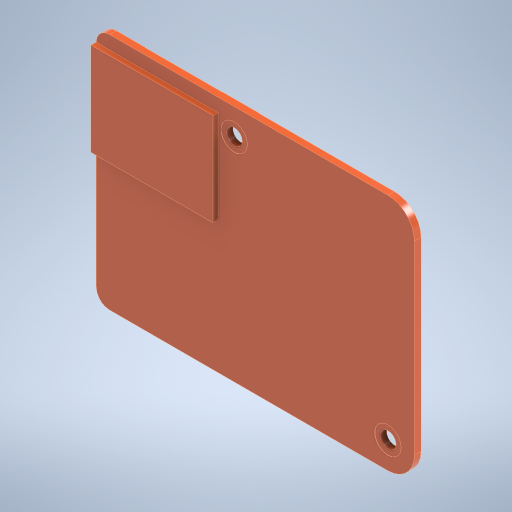
# Autodesk Inventor part: Part1
Saved by Autodesk Inventor 2023 (Build 270158000, 158)
## iProperties
Created: 2024-10-12
Part Number: Part1
Material: Phenolic Resin
Document SubType Name: Modeling
Designer: noname
Density: 1.38 g/cm^3
Appearance: Smooth - Light Orange
Mass: 5.00354 g
Surface Area: 57.0326 cm^2
Volume: 3.62576 cm^3
Author: noname
Autodesk Inventor part; units mm, degrees
ref_plane "YZ Plane" through (0, 0, 0) normal (1, 0, 0) x (0, 1, 0)
ref_plane "XZ Plane" through (0, 0, 0) normal (0, 1, 0) x (-1, 0, 0)
ref_plane "XY Plane" through (0, 0, 0) normal (0, 0, 1) x (1, 0, 0)
sketch "Sketch1" plane through (0, 0, 0) normal (0, 0, 1) x (1, 0, 0)
  line L0 (10.25, 20.1716) -> (10.25, 23.6716) projected
  line L1 (-1.25, 23.6716) -> (10.25, 23.6716) projected
  arc A0 (0.75, 23.3284) -> (-1.25, 23.6716) centre (-1.25, 17.6716) ccw projected
  line L2 (0.75, 23.3284) -> (0.75, -11.8284) projected
  arc A1 (-1.25, -13.8284) -> (0.75, -11.8284) centre (-1.25, -11.8284) ccw projected
  arc A2 (-1.25, -13.8284) -> (-4.75, -17.3284) centre (-1.25, -17.3284) ccw projected
  line L3 (-4.75, -17.3284) -> (-4.75, -23.3284) projected
  line L4 (10.25, -23.3284) -> (-4.75, -23.3284) projected
  line L5 (10.25, -23.3284) -> (10.25, -19.8284) projected
  line L6 (10.25, -19.8284) -> (6.75, -19.8284) projected
  line L7 (6.75, -19.8284) -> (6.75, 8.1716) projected
  line L8 (6.75, 8.1716) -> (16.75, 8.1716) projected
  line L9 (16.75, 17.1716) -> (16.75, 8.1716) projected
  line L10 (16.75, 17.1716) -> (13.25, 17.1716) projected
  arc A3 (10.25, 20.1716) -> (13.25, 17.1716) centre (13.25, 20.1716) ccw projected
  circle A4 centre (-1.25, -17.3284) radius 1.5 projected
  line L11 (-57.25, 4.6716) -> (-57.25, 20.1716) projected
  line L12 (-57.25, 4.6716) -> (-50.25, 4.6716) projected
  arc A5 (-50.25, 4.6716) -> (-48.25, 6.6716) centre (-50.25, 6.6716) ccw projected
  line L13 (-48.25, 6.6716) -> (-48.25, 23.6716) projected
  line L14 (-53.75, 23.6716) -> (-48.25, 23.6716) projected
  arc A6 (-53.75, 23.6716) -> (-57.25, 20.1716) centre (-53.75, 20.1716) ccw projected
  line L15 (-26.75, 17.6716) -> (-26.75, 23.6716) projected
  line L16 (-33.75, 23.6716) -> (-26.75, 23.6716) projected
  line L17 (-33.75, 23.6716) -> (-33.75, 17.6716) projected
  arc A7 (-33.75, 17.6716) -> (-26.75, 17.6716) centre (-30.25, 17.6716) ccw projected
  circle A8 centre (-30.25, 17.6716) radius 1.5 projected
  line L18 (-50.25, 4.6716) -> (-57.25, 4.6716) projected
  line L19 (-57.25, -19.8284) -> (-57.25, 4.6716) projected
  arc A9 (-57.25, -19.8284) -> (-53.75, -23.3284) centre (-53.75, -19.8284) ccw projected
  line L20 (-4.75, -23.3284) -> (-53.75, -23.3284) projected
  line L21 (-4.75, -23.3284) -> (-4.75, -17.3284) projected
  arc A10 (-1.25, -13.8284) -> (-4.75, -17.3284) centre (-1.25, -17.3284) ccw projected
  arc A11 (-1.25, -13.8284) -> (0.75, -11.8284) centre (-1.25, -11.8284) ccw projected
  line L22 (0.75, -11.8284) -> (0.75, 23.3284) projected
  arc A12 (0.75, 23.3284) -> (-1.25, 23.6716) centre (-1.25, 17.6716) ccw projected
  line L23 (-26.75, 23.6716) -> (-1.25, 23.6716) projected
  line L24 (-26.75, 23.6716) -> (-26.75, 17.6716) projected
  arc A13 (-33.75, 17.6716) -> (-26.75, 17.6716) centre (-30.25, 17.6716) ccw projected
  line L25 (-33.75, 17.6716) -> (-33.75, 23.6716) projected
  line L26 (-48.25, 23.6716) -> (-33.75, 23.6716) projected
  line L27 (-48.25, 23.6716) -> (-48.25, 6.6716) projected
  arc A14 (-50.25, 4.6716) -> (-48.25, 6.6716) centre (-50.25, 6.6716) ccw projected
  line L28 (-1.25, -17.3284) -> (-53.75, -17.3284) construction
  line L29 (-53.75, -17.3284) -> (-53.75, 20.1716) construction
  line L30 (-53.75, 20.1716) -> (-1.25, 20.1716) construction
  line L31 (-1.25, 20.1716) -> (-1.25, -17.3284) construction
  arc A15 (-1.25, -22.3284) -> (3.75, -17.3284) centre (-1.25, -17.3284) ccw
  line L32 (-1.25, -22.3284) -> (-4.75, -22.3284)
  line L33 (3.75, -17.3284) -> (3.75, 17.6716)
  arc A16 (3.75, 17.6716) -> (0.75, 22.2541) centre (-1.25, 17.6716) ccw
  line L34 (-56.25, 4.6716) -> (-56.25, 20.1716)
  line L35 (-48.25, 22.6716) -> (-53.75, 22.6716)
  arc A17 (-53.75, 22.6716) -> (-56.25, 20.1716) centre (-53.75, 20.1716) ccw
  line L36 (-26.75, 22.6716) -> (-33.75, 22.6716)
  point P0 (0, 0)
  dimension "d0" = 5
  dimension "d1" = 2.5
  constraints: 18 end point, 6 point on circle, 6 point on line, 5 tangent, 4 perpendicular, 3 centre point, 3 coincident, 2 horizontal, 2 parallel, 1 horizontal alignment, 1 vertical
  measures "d0" radius of A15
  measures "d1" radius of A17
extrude "Extrusion1" add sketch "Sketch1" along normal blind 0.05 contours A16 L33 A15 L32 L3 A2 A1 L2 | L15 A7 L17 L36 | L13 A5 L12 L34 A17 L35
sketch "Sketch2" plane through (0, 0, 0.05) normal (0, 0, 1) x (1, 0, 0)
  arc A0 (3.75, 17.6716) -> (0.75, 22.2541) centre (-1.25, 17.6716) ccw projected
  line L0 (0.75, 22.2541) -> (0.75, -11.8284) projected
  arc A1 (-1.25, -13.8284) -> (0.75, -11.8284) centre (-1.25, -11.8284) ccw projected
  arc A2 (-1.25, -13.8284) -> (-4.75, -17.3284) centre (-1.25, -17.3284) ccw projected
  line L1 (-4.75, -17.3284) -> (-4.75, -22.3284) projected
  line L2 (-4.75, -22.3284) -> (-1.25, -22.3284) projected
  arc A3 (-1.25, -22.3284) -> (3.75, -17.3284) centre (-1.25, -17.3284) ccw projected
  line L3 (3.75, -17.3284) -> (3.75, 17.6716) projected
  circle A4 centre (-1.25, -17.3284) radius 1.5 projected
  line L4 (-56.25, 20.1716) -> (-56.25, 4.6716) projected
  line L5 (-56.25, 4.6716) -> (-50.25, 4.6716) projected
  arc A5 (-50.25, 4.6716) -> (-48.25, 6.6716) centre (-50.25, 6.6716) ccw projected
  line L6 (-48.25, 6.6716) -> (-48.25, 22.6716) projected
  line L7 (-48.25, 22.6716) -> (-53.75, 22.6716) projected
  arc A6 (-53.75, 22.6716) -> (-56.25, 20.1716) centre (-53.75, 20.1716) ccw projected
  arc A7 (0.75, 22.2541) -> (-1.25, 22.6716) centre (-1.25, 17.6716) ccw
  line L8 (-1.25, 22.6716) -> (-48.25, 22.6716)
  arc A8 (-57.1041, -20.8284) -> (-53.75, -23.3284) centre (-53.75, -19.8284) ccw projected
  arc A9 (-56.25, -19.8284) -> (-53.75, -22.3284) centre (-53.75, -19.8284) ccw
  line L9 (-4.75, -22.3284) -> (-53.75, -22.3284)
  line L10 (-56.25, -19.8284) -> (-56.25, 4.6716)
  circle A10 centre (-30.25, 17.6716) radius 1.5 projected
  point P0 (0, 0)
  constraints: 7 end point, 4 point on circle, 2 centre point, 2 coincident, 2 collinear, 1 horizontal, 1 tangent
extrude "Extrusion2" add sketch "Sketch2" along normal blind 1.2
sketch "Sketch3" plane through (0, 0, 1.25) normal (0, 0, 1) x (1, 0, 0)
  arc A0 (-56.25, -19.8284) -> (-53.75, -22.3284) centre (-53.75, -19.8284) ccw projected
  line L0 (-53.75, -22.3284) -> (-1.25, -22.3284) projected
  arc A1 (-1.25, -22.3284) -> (3.75, -17.3284) centre (-1.25, -17.3284) ccw projected
  line L1 (3.75, -17.3284) -> (3.75, 17.6716) projected
  arc A2 (3.75, 17.6716) -> (-1.25, 22.6716) centre (-1.25, 17.6716) ccw projected
  line L2 (-1.25, 22.6716) -> (-53.75, 22.6716) projected
  arc A3 (-53.75, 22.6716) -> (-56.25, 20.1716) centre (-53.75, 20.1716) ccw projected
  line L3 (-56.25, 20.1716) -> (-56.25, -19.8284) projected
  circle A4 centre (-1.25, -17.3284) radius 1.5 projected
  circle A5 centre (-30.25, 17.6716) radius 1.5 projected
  circle A6 centre (-1.25, -17.3284) radius 1.5 projected
  circle A7 centre (-1.25, -17.3284) radius 2.5
  circle A8 centre (-30.25, 17.6716) radius 2.5
  point P0 (0, 0)
  dimension "d6" = 5
  dimension "d7" = 5
  constraints: 2 centre point, 2 coincident
  measures "d6" diameter of A7
  measures "d7" diameter of A8
extrude "Extrusion3" cut sketch "Sketch3" against normal blind 0.05 contours A4 | A5 | A7 | A8
sketch "Sketch4" plane through (0, 0, 1.25) normal (0, 0, 1) x (1, 0, 0)
  line L0 (-56.25, 20.1716) -> (-56.25, -19.8284) projected
  line L1 (-56.25, 20.1716) -> (-33.25, 20.1716)
  line L2 (-33.25, 20.1716) -> (-33.25, 2.6716)
  line L3 (-33.25, 2.6716) -> (-56.25, 2.6716)
  line L4 (-56.25, 2.6716) -> (-56.25, 20.1716)
  point P0 (0, 0)
  point P1 (-56.25, 2.6716)
  dimension "d10" = 17.5
  dimension "d11" = 23
  constraints: 8 end point, 2 parallel, 1 horizontal, 1 perpendicular
  measures "d10" distance between parallel lines of L1 L3
  measures "d11" distance between parallel lines of L0 L2
extrude "Extrusion4" add sketch "Sketch4" along normal blind 1
body "Solid1"
